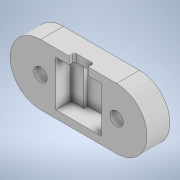
# Autodesk Inventor part: LenkwinkelsensorAS5600
Saved by Autodesk Inventor 2021 (Build 250183000, 183)
## iProperties
Created: 2021-07-19
Part Number: LenkwinkelsensorAS5600
Material: Generisch
Document SubType Name: Modeling
Designer: Lars-Ole
Density: 1 g/cm^3
Appearance: Vorgabe
Author: Lars-Ole
Autodesk Inventor part; units mm, degrees
ref_plane "YZ Plane" through (0, 0, 0) normal (1, 0, 0) x (0, 1, 0)
ref_plane "XZ Plane" through (0, 0, 0) normal (0, 1, 0) x (-1, 0, 0)
ref_plane "XY Plane" through (0, 0, 0) normal (0, 0, 1) x (1, 0, 0)
sketch "Skizze1" plane through (0, 0, 0) normal (0, 0, 1) x (1, 0, 0)
  line L0 (10, 0) -> (-10, 0) construction
  line L1 (10, 8) -> (-10, 8)
  line L2 (-10, -8) -> (10, -8)
  arc A0 (10, -8) -> (10, 8) centre (10, 0) ccw
  arc A1 (-10, 8) -> (-10, -8) centre (-10, 0) ccw
  circle A2 centre (-10, 0) radius 1.75
  circle A3 centre (10, 0) radius 1.75
  point P0 (0, 0)
  dimension "d0" = 16
  dimension "d1" = 20
  dimension "d2" = 3.5
  dimension "d3" = 3.5
  constraints: 8 end point, 4 centre point, 4 point on circle, 4 tangent, 2 coincident, 1 horizontal, 1 midpoint, 1 parallel
  measures "d0" distance between parallel lines of L2 L1
  measures "d1" distance of L0.start L0.end
  measures "d2" diameter of A2
  measures "d3" diameter of A3
extrude "Extrusion1" add sketch "Skizze1" along normal blind 6
sketch "Skizze2" plane through (0, 0, 6) normal (0, 0, 1) x (1, 0, 0)
  line L0 (6, -6) -> (-6, -6)
  line L1 (-6, -6) -> (-6, 6)
  line L2 (-6, 6) -> (6, 6)
  line L3 (6, 6) -> (6, -6)
  line L4 (6, -6) -> (-6, 6) construction
  line L5 (-6, -6) -> (6, 6) construction
  point P0 (0, 0)
  dimension "d6" = 12
  dimension "d7" = 12
  constraints: 12 end point, 2 midpoint, 2 parallel, 1 horizontal, 1 perpendicular
  measures "d6" distance of L1.end L2.end
  measures "d7" distance of L0.end L1.end
extrude "Extrusion2" cut sketch "Skizze2" against normal blind 4
sketch "Skizze3" plane through (-10, 8, 0) normal (0, 1, 0) x (1, 0, 0)
  line L0 (10, 1.2) -> (10, -7.2) projected
  line L1 (4, -6) -> (16, -6) projected
  line L2 (12.5, -4.5) -> (7.5, -4.5)
  line L3 (7.5, -4.5) -> (7.5, -6)
  line L4 (7.5, -6) -> (12.5, -6)
  line L5 (12.5, -6) -> (12.5, -4.5)
  line L6 (12.5, -4.5) -> (7.5, -6) construction
  line L7 (7.5, -4.5) -> (12.5, -6) construction
  point P0 (10, -5.25)
  dimension "d10" = 5
  dimension "d11" = 1.5
  constraints: 12 end point, 2 midpoint, 2 parallel, 2 point on line, 1 horizontal, 1 perpendicular
  measures "d10" distance of L2.start L2.end
  measures "d11" distance of L2.end L3.end
extrude "Extrusion3" cut sketch "Skizze3" against normal up to next
fillet "Rundung1" radius 0.5 2 edges at (-2.5, 7, 4.5) (2.5, 7, 4.5)
sketch "Skizze4" plane through (0, 0, 2) normal (0, 0, 1) x (1, 0, 0)
  line L0 (2.6, -6) -> (-2.6, -6)
  line L1 (-2.6, -6) -> (-2.6, 6)
  line L2 (-2.6, 6) -> (2.6, 6)
  line L3 (2.6, 6) -> (2.6, -6)
  line L4 (2.6, -6) -> (-2.6, 6) construction
  line L5 (-2.6, -6) -> (2.6, 6) construction
  line L6 (6, -6) -> (-6, -6) projected
  point P0 (0, 0)
  dimension "d15" = 5.2
  constraints: 12 end point, 2 midpoint, 2 parallel, 1 horizontal, 1 perpendicular, 1 point on line
  measures "d15" distance of L1.end L2.end
extrude "Extrusion4" cut sketch "Skizze4" against normal blind 1
equation "\"d3\" = d2"
